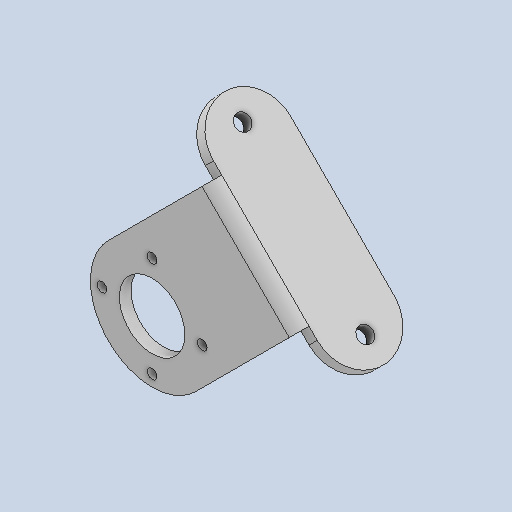
# Autodesk Inventor part: Uchwyt_silnika_1
Saved by Autodesk Inventor 2022.3 (Build 263350000, 350)
## iProperties
Created: 2023-01-03
Part Number: Uchwyt_silnika_1
Material: Generic
Document SubType Name: Sheet Metal
Designer: komputer
Density: 1 g/cm^3
Appearance: Default
Sheet Metal Rule: Default_mm
Author: komputer
Autodesk Inventor part; units mm, degrees
ref_plane "YZ Plane" through (0, 0, 0) normal (1, 0, 0) x (0, 1, 0)
ref_plane "XZ Plane" through (0, 0, 0) normal (0, 1, 0) x (-1, 0, 0)
ref_plane "XY Plane" through (0, 0, 0) normal (0, 0, 1) x (1, 0, 0)
sketch "Sketch1" plane through (0, 0, 0) normal (0, 0, 1) x (1, 0, 0)
  circle A0 centre (0, 0) radius 16 projected
  circle A1 centre (-13, 0) radius 1.25 projected
  circle A2 centre (0, -13) radius 1.25 projected
  circle A3 centre (13, 0) radius 1.25 projected
  circle A4 centre (0, 13) radius 1.25 projected
  circle A5 centre (0, 0) radius 8.5 projected
  line L0 (-13, 0) -> (0, -13)
  line L1 (0, -13) -> (13, 0)
  line L2 (13, 0) -> (0, 13)
  line L3 (0, 13) -> (-13, 0)
  circle A6 centre (0, 0) radius 16
  line L4 (-11.3137, 11.3137) -> (3.9161, 26.5436)
  line L5 (11.3137, -11.3137) -> (26.5436, 3.9161)
  line L6 (11.3137, 11.3137) -> (-3.2223, 25.8497)
  line L7 (-3.2223, 25.8497) -> (25.9716, -3.3441)
  line L8 (0, 22.6274) -> (10.6066, 33.234)
  line L9 (22.6274, 0) -> (33.234, 10.6066)
  line L10 (33.234, 10.6066) -> (10.6066, 33.234)
  point P0 (0, 0)
  dimension "d0" = 15
  dimension "d1" = 15
  constraints: 22 end point, 7 point on line, 6 tangent, 3 parallel, 3 perpendicular, 3 point on circle, 1 centre point, 1 coincident, 1 concentric
  measures "d0" distance of L8.start L8.end
  measures "d1" distance of L9.start L9.end
extrude "Extrusion1" add sketch "Sketch1" along normal blind 3 contours A0 | A0 L7 L5 | A0 L4 L6 | L6 L4 L8 L10 L9 L5 L7 | A1 L3 A4 L2 A3 L1 A2 L0
sketch "Sketch2" plane through (0, 0, 3) normal (0, 0, 1) x (1, 0, 0)
  line L0 (10.6066, 33.234) -> (-11.3137, 11.3137) projected
  arc A0 (-11.3137, 11.3137) -> (11.3137, -11.3137) centre (0, 0) ccw projected
  line L1 (11.3137, -11.3137) -> (33.234, 10.6066) projected
  line L2 (33.234, 10.6066) -> (10.6066, 33.234) projected
  circle A1 centre (13, 0) radius 1.25 projected
  circle A2 centre (0, -13) radius 1.25 projected
  circle A3 centre (-13, 0) radius 1.25 projected
  circle A4 centre (0, 0) radius 8.5 projected
  circle A5 centre (0, 13) radius 1.25 projected
  circle A6 centre (-13, 0) radius 1.25 projected
  circle A7 centre (0, 13) radius 1.25 projected
  line L3 (-13, 0) -> (0, 13)
  circle A8 centre (0, -13) radius 1.25 projected
  circle A9 centre (13, 0) radius 1.25 projected
  line L4 (0, -13) -> (13, 0)
  circle A10 centre (0, 0) radius 8.5 projected
  line L5 (0, 0) -> (28.2843, 28.2843)
  line L6 (-13, 0) -> (0, -13)
  line L7 (33.234, 10.6066) -> (10.6066, 33.234) projected
  line L8 (10.6066, 33.234) -> (35.7367, 58.3641)
  line L9 (33.234, 10.6066) -> (59.3246, 36.6972)
  line L10 (11.3137, -11.3137) -> (33.234, 10.6066) projected
  line L11 (10.6066, 33.234) -> (-11.3137, 11.3137) projected
  line L12 (28.2843, 28.2843) -> (39.598, 16.9706)
  line L13 (28.2843, 28.2843) -> (16.9706, 39.598)
  point P0 (0, 0)
  dimension "d4" = 40
  constraints: 16 end point, 4 parallel, 3 perpendicular, 3 point on line, 2 collinear
  measures "d4" distance of L5.start L5.end
extrude "Extrusion2" add sketch "Sketch2" against normal up to surface (3 mm away) contours L8 L13 L5 L2 | L5 L12 L9 L2
sketch "Sketch3" plane through (0, 0, 0) normal (0, 0, -1) x (-1, 0, 0)
  line L0 (-16.9706, 39.598) -> (11.3137, 11.3137) projected
  line L1 (-16.9706, 39.598) -> (-39.598, 16.9706) projected
  line L2 (-11.3137, -11.3137) -> (-39.598, 16.9706) projected
  arc A0 (-11.3137, -11.3137) -> (11.3137, 11.3137) centre (0, 0) ccw projected
  circle A1 centre (-13, 0) radius 1.25 projected
  circle A2 centre (0, -13) radius 1.25 projected
  circle A3 centre (13, 0) radius 1.25 projected
  circle A4 centre (0, 0) radius 8.5 projected
  circle A5 centre (0, 13) radius 1.25 projected
  line L3 (-11.3137, -11.3137) -> (-39.598, 16.9706) projected
  line L4 (-39.598, 16.9706) -> (-37.4767, 14.8492)
  line L5 (-37.4767, 14.8492) -> (-14.8492, 37.4767)
  line L6 (-16.9706, 39.598) -> (11.3137, 11.3137) projected
  point P0 (0, 0)
  dimension "d7" = 3
  constraints: 4 end point, 2 point on line, 1 perpendicular
  measures "d7" distance of L1.end L4.end
extrude "Extrusion3" add sketch "Sketch3" along normal blind 20 contours L0 L5 L2 L1
sketch "Sketch4" plane through (39.598, 16.9706, -20) normal (0.7071068, 0.7071068, 0) x (-0.7071068, 0.7071068, 0)
  line L0 (0, 23) -> (0, 0) projected
  line L1 (32, 0) -> (0, 0) projected
  line L2 (32, 23) -> (32, 0) projected
  line L3 (32, 20) -> (32, 0) projected
  line L4 (32, 0) -> (35, 0)
  line L5 (35, 0) -> (35, 20)
  line L6 (35, 20) -> (32, 20)
  line L7 (32, 20) -> (32, 0)
  line L8 (0, 20) -> (0, 0) projected
  line L9 (0, 0) -> (-3, 0)
  line L10 (-3, 0) -> (-3, 20)
  line L11 (-3, 20) -> (0, 20)
  line L12 (0, 20) -> (0, 0)
  circle A0 centre (35, 10) radius 10
  circle A1 centre (-3, 10) radius 10
  line L13 (35, 10) -> (45, 10)
  circle A2 centre (40, 10) radius 2
  line L14 (16, 20) -> (16, 0)
  line L15 (0, 0) -> (32, 0) projected
  circle A3 centre (16, 10) radius 2
  circle A4 centre (-8, 10) radius 2
  line L16 (0, 23) -> (32, 23) projected
  point P0 (32, 19)
  point P1 (-3, 0)
  point P2 (35, 0)
  dimension "d12" = 3
  dimension "d13" = 3
  dimension "d14" = 4
  dimension "d15" = 4
  constraints: 20 end point, 5 midpoint, 4 centre point, 4 parallel, 3 horizontal, 2 perpendicular, 2 point on circle, 1 point on line, 1 symmetric about line, 4 other
  measures "d12" distance of L3.start L5.end
  measures "d13" distance of L10.end L11.end
  measures "d14" diameter of A2
  measures "d15" diameter of A3
extrude "Extrusion4" add sketch "Sketch4" against normal blind 3 contours L0 A1 L11 | L0 A1 L10 | L10 A1 | L6 A0 L2 | L0 L9 A1 | A0 L5 L2 | A0 L13 A2 L5 | A0 L4 L2 | L13 A2 A0 L5
sketch "Sketch5" plane through (12.7279, 39.598, -10) normal (-0.7071068, -0.7071068, 0) x (-0.7071068, 0.7071068, 0)
  circle A0 centre (-43, 0) radius 2 projected
  circle A1 centre (5, 0) radius 2 projected
  line L0 (-3, -10) -> (0, -10) projected
  arc A2 (0, -10) -> (0, 10) centre (0, 0) ccw projected
  line L1 (0, 10) -> (-38, 10) projected
  arc A3 (-38, 10) -> (-38, -10) centre (-38, 0) ccw projected
  line L2 (-38, -10) -> (-35, -10) projected
  circle A4 centre (-41.5, 29.4965) radius 2.25 projected
  circle A5 centre (3.5, 29.4965) radius 2.25 projected
  line L3 (-41.5, 29.4965) -> (-41.5, -27.5248)
  line L4 (3.5, 29.4965) -> (3.5, -58.5312)
  circle A6 centre (-41.5, 0) radius 2
  circle A7 centre (3.5, 0) radius 2
  line L5 (-3, -10) -> (-35, -10) projected
  point P0 (-19, -10)
  point P1 (4.25, 1.854)
  point P2 (4.25, -1.854)
  point P3 (-42.25, -1.854)
  point P4 (-42.25, 1.854)
  constraints: 4 end point, 2 centre point, 2 point on line, 2 vertical
extrude "Extrusion5" add sketch "Sketch5" against normal blind 3 contours A6 A0 | A1 A7
sketch "Sketch6" plane through (12.7279, 39.598, -10) normal (-0.7071068, -0.7071068, 0) x (-0.7071068, 0.7071068, 0)
  arc A0 (-42.25, -1.854) -> (-42.25, 1.854) centre (-43, 0) ccw projected
  arc A1 (-42.25, 1.854) -> (-42.25, -1.854) centre (-41.5, 0) ccw projected
  arc A2 (4.25, 1.854) -> (4.25, -1.854) centre (5, 0) ccw projected
  arc A3 (4.25, -1.854) -> (4.25, 1.854) centre (3.5, 0) ccw projected
  line L0 (-3, -10) -> (0, -10) projected
  arc A4 (0, -10) -> (0, 10) centre (0, 0) ccw projected
  line L1 (0, 10) -> (-38, 10) projected
  arc A5 (-38, 10) -> (-38, -10) centre (-38, 0) ccw projected
  line L2 (-38, -10) -> (-35, -10) projected
  circle A6 centre (-41.5, 0) radius 2
  circle A7 centre (3.5, 0) radius 2
  line L3 (-3, -10) -> (-35, -10) projected
  point P0 (-19, -10)
  point P1 (-42.25, -1.854)
  point P2 (-42.25, 1.854)
  point P3 (4.25, 1.854)
  constraints: 2 centre point, 2 coincident
extrude "Extrusion6" cut sketch "Sketch6" against normal blind 3 contours A0 A6 | A2 A7
sketch "Sketch8" plane through (0, 0, 3) normal (0, 0, 1) x (1, 0, 0)
  line L0 (16.9706, 39.598) -> (-11.3137, 11.3137) projected
  arc A0 (-11.3137, 11.3137) -> (11.3137, -11.3137) centre (0, 0) ccw projected
  line L1 (11.3137, -11.3137) -> (39.598, 16.9706) projected
  line L2 (39.598, 16.9706) -> (16.9706, 39.598) projected
  circle A1 centre (13, 0) radius 1.25 projected
  circle A2 centre (0, -13) radius 1.25 projected
  circle A3 centre (-13, 0) radius 1.25 projected
  circle A4 centre (0, 0) radius 8.5 projected
  circle A5 centre (0, 13) radius 1.25 projected
  circle A6 centre (-13, 0) radius 1.25 projected
  circle A7 centre (0, 13) radius 1.25 projected
  line L3 (-13, 0) -> (0, 13)
  circle A8 centre (13, 0) radius 1.25 projected
  line L4 (0, 13) -> (13, 0)
  line L5 (13, 0) -> (-0.0002, -13.0002)
  line L6 (0, 0) -> (26.3553, 26.3553)
  line L7 (26.3553, 26.3553) -> (50.7309, 1.9797)
  line L8 (14.8492, 37.4767) -> (37.4767, 14.8492) projected
  line L9 (26.3553, 26.3553) -> (4.9031, 47.8075)
  line L10 (5.6569, 46.669) -> (12.7279, 39.598) projected
  line L11 (14.8492, 37.4767) -> (20.1327, 42.7601)
  line L12 (20.1327, 42.7601) -> (7.1248, 51.3664)
  line L13 (7.1248, 51.3664) -> (0, 48.1905)
  line L14 (0, 48.1905) -> (14.8492, 37.4767)
  line L15 (11.3137, -11.3137) -> (37.4767, 14.8492) projected
  line L16 (37.4767, 14.8492) -> (41.6279, 19.0005)
  line L17 (41.6279, 19.0005) -> (52.2205, 8.9599)
  line L18 (52.2205, 8.9599) -> (46.7077, 4.5581)
  line L19 (46.7077, 4.5581) -> (37.4767, 13.3081)
  line L20 (37.4767, 13.3081) -> (37.4767, 14.8492)
  line L21 (11.3137, -11.3137) -> (39.598, 16.9706) projected
  point P0 (0, 0)
  point P1 (15.0416, 37.669)
  point P2 (37.669, 15.0416)
  dimension "d24" = 37.272
  constraints: 30 end point, 3 parallel, 3 perpendicular, 1 collinear, 1 point on line, 1 vertical
  measures "d24" distance of L6.start L6.end
extrude "Extrusion7" cut sketch "Sketch8" against normal through all contours L14 L13 L12 L11 L0 | L0 L2 L1 L7 L9 | L1 L7 L18 L19 L20 | L16 L17 L18 L7 L1
sketch "Sketch9" plane through (0, 0, 3) normal (0, 0, 1) x (1, 0, 0)
  circle A0 centre (0, 13) radius 1.25 projected
  circle A1 centre (0, 0) radius 8.5 projected
  circle A2 centre (-13, 0) radius 1.25 projected
  circle A3 centre (0, -13) radius 1.25 projected
  circle A4 centre (13, 0) radius 1.25 projected
  line L0 (37.669, 15.0416) -> (15.0416, 37.669) projected
  line L1 (15.0416, 37.669) -> (-11.3137, 11.3137) projected
  arc A5 (-11.3137, 11.3137) -> (11.3137, -11.3137) centre (0, 0) ccw projected
  line L2 (11.3137, -11.3137) -> (37.669, 15.0416) projected
  line L3 (37.669, 15.0416) -> (15.0416, 37.669) projected
  line L4 (15.0416, 37.669) -> (12.9203, 35.5477)
  line L5 (15.0416, 37.669) -> (-11.3137, 11.3137) projected
  line L6 (12.9203, 35.5477) -> (38.0462, 10.4217)
  point P0 (0, 0)
  point P1 (35.5477, 12.9203)
  dimension "d27" = 3
  constraints: 4 end point, 1 perpendicular, 1 point on line
  measures "d27" distance of L0.end L4.end
extrude "Extrusion8" add sketch "Sketch9" against normal up to surface (23 mm away) contours L2 L6 L1 L0
sketch "Sketch10" plane through (12.9203, 35.5477, 0) normal (-0.7071068, -0.7071068, 0) x (-0.7071068, 0.7071068, 0)
  circle A0 centre (6.5, 39.4965) radius 2 projected
  circle A1 centre (6.5, 10) radius 2 projected
  circle A2 centre (-38.5, 10) radius 2 projected
  line L0 (0, 0) -> (-32, 0) projected
  line L1 (0, 0) -> (0, 20) projected
  line L2 (0, 20) -> (-32, 20) projected
  line L3 (-32, 0) -> (-32, 20) projected
  line L4 (-32, 49.4965) -> (-35, 49.4965) projected
  line L5 (-32, 29.4965) -> (-32, 49.4965) projected
  line L6 (-35, 29.4965) -> (-32, 29.4965) projected
  arc A3 (-35, 49.4965) -> (-35, 29.4965) centre (-35, 39.4965) ccw projected
  circle A4 centre (-38.5, 39.4965) radius 2.25 projected
  line L7 (0, 29.4965) -> (3, 29.4965) projected
  line L8 (0, 49.4965) -> (0, 29.4965) projected
  line L9 (3, 49.4965) -> (0, 49.4965) projected
  arc A5 (3, 29.4965) -> (3, 49.4965) centre (3, 39.4965) ccw projected
  circle A6 centre (6.5, 39.4965) radius 2.25 projected
  circle A7 centre (3, 10) radius 10
  line L10 (0, 20) -> (-32, 20) projected
  line L11 (0, 20) -> (3, 20)
  line L12 (0, 0) -> (-32, 0) projected
  line L13 (0, 0) -> (3, 0)
  line L14 (-16, 20) -> (-16, 12.7343)
  circle A8 centre (-38.5, 10) radius 2
  circle A9 centre (-35, 10) radius 10
  line L15 (-32, 20) -> (-35, 20)
  line L16 (-32, 0) -> (-35, 0)
  point P0 (-16, 0)
  constraints: 10 end point, 4 point on circle, 4 symmetric about line, 3 centre point, 2 collinear, 1 midpoint, 1 vertical, 2 other
extrude "Extrusion9" add sketch "Sketch10" against normal blind 3 contours L1 A7 L13 | L16 A9 L3 | L1 A7 | A9 L3 | L1 L11 A7 | A9 L15 L3 picked at (1.5, 10) picked at (-33.5, 10)
fillet "Fillet4" radius 3 1 edges at (26.3553, 26.3553, 3)
fillet "Fillet5" radius 1 1 edges at (24.234, 24.234, 0)
equation "\"BendRadius\" = Thickness"
equation "\"BendReliefWidth\" = Thickness"
equation "\"BendReliefDepth\" = 0.5 * Thickness"
equation "\"CornerReliefSize\" = 4 * Thickness"
equation "\"MinimumRemnant\" = 2 * Thickness"
equation "\"TransitionRadius\" = BendRadius"
equation "\"JacobiRadiusSize\" = BendRadius"
equation "\"GapSize\" = Thickness"
equation "\"Thickness\" = 3.414214"
body "Solid1"
